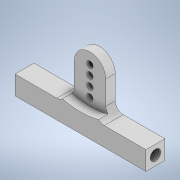
# Autodesk Inventor part: workTrianglePc1
Saved by Autodesk Inventor 2021 (Build 250183000, 183)
## iProperties
Created: 2022-09-09
Part Number: workTrianglePc1
Material: Generic
Document SubType Name: Modeling
Designer: szucs
Density: 1 g/cm^3
Appearance: Default
Author: szucs
Autodesk Inventor part; units mm, degrees
ref_plane "YZ Plane" through (0, 0, 0) normal (1, 0, 0) x (0, 1, 0)
ref_plane "XZ Plane" through (0, 0, 0) normal (0, 1, 0) x (-1, 0, 0)
ref_plane "XY Plane" through (0, 0, 0) normal (0, 0, 1) x (1, 0, 0)
sketch "Sketch1" plane through (0, 0, 0) normal (0, 0, 1) x (1, 0, 0)
  line L0 (0, 23.4) -> (0, -35.4) projected
  line L1 (-58.1, 0) -> (58.1, 0) projected
  line L2 (-10, 15) -> (10, 15)
  line L3 (10, 15) -> (10, -15)
  line L4 (10, -15) -> (-10, -15)
  line L5 (-10, -15) -> (-10, 15)
  line L6 (-41.5, -15) -> (41.5, -15)
  line L7 (41.5, -15) -> (41.5, -27)
  line L8 (41.5, -27) -> (-41.5, -27)
  line L9 (-41.5, -27) -> (-41.5, -15)
  point P0 (0, 0)
  point P1 (10, -15)
  point P2 (-10, -15)
  dimension "d0" = 30
  dimension "d1" = 12
  dimension "d2" = 83
  dimension "d3" = 20
  constraints: 16 end point, 4 parallel, 2 horizontal, 2 perpendicular, 1 point on line, 3 other
  measures "d0" distance of L2.end L3.end
  measures "d1" distance of L8.end L6.start
  measures "d2" distance of L7.end L8.end
  measures "d3" distance between parallel lines of L5 L3
extrude "Extrusion1" add sketch "Sketch1" along normal blind 12
sketch "Sketch2" plane through (41.5, -27, 0) normal (1, 0, 0) x (0, 0, -1)
  line L0 (0, 12) -> (-12, 12) projected
  line L1 (-12, 0) -> (-12, 12) projected
  point P0 (0, 27)
  point P1 (-6, 6)
  dimension "d6" = 6
  dimension "d7" = 6
  measures "d6" distance from line of L0 point (-6, 6)
  measures "d7" distance from line of L1 point (-6, 6)
hole "Hole1" at (41.5, -21, 6) direction (-1, 0, 0) diameter 6.647 depth 35 tip angle 118 thread size "M8x1.25" class "6H" standard "ISO Metric profile"
sketch "Sketch3" plane through (-41.5, -27, 0) normal (-1, 0, 0) x (0, 0, 1)
  line L0 (0, 12) -> (12, 12) projected
  line L1 (0, 12) -> (0, 0) projected
  point P0 (0, 27)
  point P1 (6, 6)
  dimension "d15" = 6
  dimension "d16" = 6
  measures "d15" distance from line of L0 point (6, 6)
  measures "d16" distance from line of L1 point (6, 6)
hole "Hole2" at (-41.5, -21, 6) direction (1, 0, 0) diameter 6.647 depth 35 tip angle 118 thread size "M8x1.25" class "6H" standard "ISO Metric profile"
sketch "Sketch4" plane through (0, 0, 12) normal (0, 0, 1) x (1, 0, 0)
  line L0 (-10, 15) -> (-10, -15) projected
  line L1 (-10, -15) -> (-41.5, -15) projected
  line L2 (-41.5, -15) -> (-41.5, -27) projected
  line L3 (-41.5, -27) -> (41.5, -27) projected
  line L4 (41.5, -27) -> (41.5, -15) projected
  line L5 (41.5, -15) -> (10, -15) projected
  line L6 (10, -15) -> (10, 15) projected
  circle A0 centre (0, -10) radius 2
  line L7 (10, 15) -> (-10, 15) projected
  circle A1 centre (0, -4) radius 2
  circle A2 centre (0, 2) radius 2
  circle A3 centre (0, 8) radius 2
  point P0 (0, 0)
  dimension "d26" = 4
  dimension "d50" = 17
  dimension "d51" = 10
  dimension "d52" = 4
  dimension "d53" = 6
  dimension "d54" = 4
  dimension "d55" = 10
  dimension "d56" = 6
  dimension "d57" = 10
  dimension "d58" = 4
  dimension "d59" = 10
  dimension "d60" = 6
  constraints: 4 centre point
  measures "d26" diameter of A0
  measures "d50" distance from line of L3 A0.centre
  measures "d51" distance from line of L0 A0.centre
  measures "d52" diameter of A1
  measures "d53" distance of A1.centre A0.centre
  measures "d54" diameter of A2
  measures "d55" distance from line of L0 A1.centre
  measures "d56" distance of A2.centre A1.centre
  measures "d57" distance from line of L6 A2.centre
  measures "d58" diameter of A3
  measures "d59" distance from line of L6 A3.centre
  measures "d60" distance of A2.centre A3.centre
extrude "Extrusion2" cut sketch "Sketch4" against normal through all contours A0 | A1 | A2 | A3
fillet "Fillet2" radius 5 2 edges at (10, -15, 6) (-10, -15, 6)
sketch "Sketch5" plane through (0, 0, 12) normal (0, 0, 1) x (1, 0, 0)
  line L0 (-10, 15) -> (-10, -10) projected
  arc A0 (-15, -15) -> (-10, -10) centre (-15, -10) ccw projected
  line L1 (-15, -15) -> (-41.5, -15) projected
  line L2 (-41.5, -15) -> (-41.5, -27) projected
  line L3 (-41.5, -27) -> (41.5, -27) projected
  line L4 (41.5, -27) -> (41.5, -15) projected
  line L5 (41.5, -15) -> (15, -15) projected
  arc A1 (10, -10) -> (15, -15) centre (15, -10) ccw projected
  line L6 (10, -10) -> (10, 15) projected
  circle A2 centre (0, -10) radius 2 projected
  line L7 (-54.6159, 30) -> (65.6495, 30)
  line L8 (0, 98.4) -> (0, -47.9) projected
  circle A3 centre (0, 30) radius 45
  line L9 (10, 15) -> (-10, 15) projected
  circle A4 centre (0, 8) radius 2 projected
  point P0 (0, 0)
  point P1 (-11.4484, -13.5194)
  point P2 (11.4484, -13.5194)
  point P3 (10.181, -11.3332)
  point P4 (-10.181, -11.3332)
  dimension "d42" = 57
  dimension "d43" = 90
  constraints: 2 end point, 2 point on line, 1 centre point, 1 horizontal
  measures "d42" distance between parallel lines of L3 L7
  measures "d43" diameter of A3
extrude "Extrusion3" cut sketch "Sketch5" against normal blind 6 contours L9 L8 A4 A2 A3 A0 L0 | L0 A0 A3 L7 L8 L9 | L9 L6 A1 A3 L8 A2 A4 | L8 L7 A3 A1 L6 L9 | L8 A3 L7 | L7 A3 L8 | A4 L8 | L8 A4
fillet "Fillet4" radius 10 2 edges at (10, 15, 3) (-10, 15, 3)
body "Solid1"
